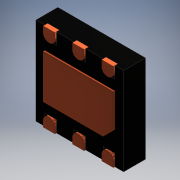
# Autodesk Inventor part: 3x3 6-pin DFN
Saved by Autodesk Inventor 2016 (Build 200138000, 138)
## iProperties
Created: 2016-07-18
Part Number: 3x3 6-pin DFN
Material: Generic
Document SubType Name: Modeling
Designer: Jonathan
Density: 1 g/cm^3
Appearance: Default
Author: Jonathan
Autodesk Inventor part; units mm, degrees
ref_plane "YZ Plane" through (0, 0, 0) normal (1, 0, 0) x (0, 1, 0)
ref_plane "XZ Plane" through (0, 0, 0) normal (0, 1, 0) x (-1, 0, 0)
ref_plane "XY Plane" through (0, 0, 0) normal (0, 0, 1) x (1, 0, 0)
sketch "Sketch1" plane through (0, 0, 0) normal (0, 1, 0) x (-1, 0, 0)
  line L0 (-1.5, 1.5) -> (1.5, 1.5)
  line L1 (1.5, 1.5) -> (1.5, -1.5)
  line L2 (1.5, -1.5) -> (-1.5, -1.5)
  line L3 (-1.5, -1.5) -> (-1.5, 1.5)
  line L4 (-1.5, 1.5) -> (1.5, -1.5) construction
  line L5 (1.5, 1.5) -> (-1.5, -1.5) construction
  point P0 (0, 0)
  dimension "d0" = 3
  dimension "d1" = 3
  constraints: 12 end point, 2 midpoint, 2 parallel, 1 horizontal, 1 perpendicular
  measures "d0" distance of L0.end L1.end
  measures "d1" distance of L0.start L0.end
extrude "Extrusion1" add sketch "Sketch1" along normal mid plane 0.75
sketch "Sketch3" plane through (0, -0.375, 0) normal (0, -1, 0) x (1, 0, 0)
  line L0 (-1.5, 1.5) -> (1.5, 1.5) projected
  line L1 (0.2, 1.5) -> (-0.2, 1.5)
  line L2 (-0.2, 1.5) -> (-0.2, 1.1)
  line L3 (-0.2, 1.1) -> (0.2, 1.1)
  line L4 (0.2, 1.1) -> (0.2, 1.5)
  point P0 (0, 0)
  point P1 (0, 1.1)
  dimension "d6" = 0.4
  dimension "d7" = 0.4
  constraints: 8 end point, 2 parallel, 1 horizontal, 1 midpoint, 1 perpendicular, 1 point on line, 1 vertical alignment
  measures "d6" distance of L3.end L1.start
  measures "d7" distance of L2.end L3.end
extrude "Extrusion2" cut sketch "Sketch3" against normal blind 0.1
sketch "Sketch4" plane through (0, -0.275, 0) normal (0, -1, 0) x (1, 0, 0)
  line L0 (-0.2, 1.1) -> (-0.2, 1.5) projected
  line L1 (0.2, 1.5) -> (-0.2, 1.5)
  line L2 (-0.2, 1.5) -> (-0.2, 1.4)
  line L3 (-0.2, 1.4) -> (0.2, 1.4)
  line L4 (0.2, 1.4) -> (0.2, 1.5)
  line L5 (0.2, 1.5) -> (0.2, 1.1) projected
  point P0 (0, 0)
  dimension "d10" = 0.1
  constraints: 8 end point, 2 parallel, 1 collinear, 1 horizontal, 1 perpendicular, 1 point on line
  measures "d10" distance of L3.end L1.start
extrude "Extrusion3" add sketch "Sketch4" along normal blind 0.15 separate body
sketch "Sketch6" plane through (0, -0.425, 0) normal (0, -1, 0) x (1, 0, 0)
  line L0 (-0.2, 1.4) -> (0.2, 1.4) projected
  line L1 (0.2, 1.4) -> (0.2, 1.3)
  line L2 (-0.2, 1.4) -> (-0.2, 1.3)
  line L3 (-0.2, 1.1) -> (-0.2, 1.5) projected
  arc A0 (-0.2, 1.3) -> (0.2, 1.3) centre (0, 1.3) ccw
  line L4 (0.25, 1.1) -> (-0.25, 1.1) construction
  line L5 (0.2, 1.1) -> (-0.2, 1.1) projected
  point P0 (0, 0)
  point P1 (0, 1.1)
  dimension "d13" = 0.5
  constraints: 6 end point, 3 point on circle, 2 midpoint, 2 tangent, 1 centre point, 1 collinear, 1 horizontal, 1 vertical
  measures "d13" distance of L4.start L4.end
extrude "Extrusion4" add sketch "Sketch6" against normal blind 0.1 contours L0 L1 A0 L2 bodies 2
pattern_linear "Rectangular Pattern1" count 2 spacing 1 along (-1, 0, 0) count 2 spacing 1 along (1, 0, 0) of "Extrusion2" bodies 1
pattern_linear "Rectangular Pattern2" count 2 spacing 1 along (-1, 0, 0) count 2 spacing 1 along (1, 0, 0) of "Extrusion3", "Extrusion4" bodies 2
mirror "Mirror1" about plane through (0, 0, 0) normal (0, 0, 1) of "Extrusion2", "Rectangular Pattern1" bodies 1
mirror "Mirror2" about plane through (0, 0, 0) normal (0, 0, 1) of "Extrusion3", "Extrusion4", "Rectangular Pattern2" bodies 2
sketch "Sketch7" plane through (0, -0.375, 0) normal (0, -1, 0) x (1, 0, 0)
  line L0 (-1.2, 0.75) -> (1.2, 0.75)
  line L1 (1.2, 0.75) -> (1.2, -0.3964)
  line L2 (0.8464, -0.75) -> (-1.2, -0.75)
  line L3 (-1.2, -0.75) -> (-1.2, 0.75)
  line L4 (-1.2, 0.75) -> (1.2, -0.75) construction
  line L5 (1.2, 0.75) -> (-1.2, -0.75) construction
  line L6 (1.2, -0.3964) -> (0.8464, -0.75)
  point P0 (0, 0)
  point P1 (-0.1768, -0.75)
  point P2 (1.2, 0.1768)
  dimension "d28" = 1.5
  dimension "d29" = 2.4
  dimension "d30" = 135
  dimension "d31" = 0.5
  constraints: 14 end point, 4 midpoint, 2 parallel, 1 horizontal, 1 horizontal alignment, 1 perpendicular, 1 vertical alignment
  measures "d28" distance between parallel lines of L2 L0
  measures "d29" distance of L0.start L0.end
  measures "d30" angle of L2 L6
  measures "d31" distance of L1.end L2.start
extrude "Extrusion5" cut sketch "Sketch7" against normal blind 0.01 bodies 1
extrude "Extrusion6" add sketch "Sketch7" along normal up to surface (0.05 mm away) bodies 2
sketch "Sketch8" plane through (0, 0.375, 0) normal (0, 1, 0) x (1, 0, 0)
  circle A0 centre (0, 0) radius 0.72
  dimension "d36" = 1.44
  constraints: 1 centre point, 1 coincident
  measures "d36" diameter of A0
sketch "Sketch9" plane through (0, 0, 0) normal (0, 1, 0) x (-1, 0, 0)
  circle A0 centre (0, 0) radius 0.45
  dimension "d37" = 0.9
  constraints: 1 centre point, 1 coincident
  measures "d37" diameter of A0
loft "Loft1" cut profiles "Sketch8", "Sketch9" bodies 1
sketch "Sketch10" plane through (0, 0.375, 0) normal (0, 1, 0) x (1, 0, 0)
  circle A0 centre (1.15, 1.15) radius 0.125
  line L0 (1.5, -1.5) -> (1.5, 1.5) projected
  line L1 (1.5, 1.5) -> (-1.5, 1.5) projected
  point P0 (0, 0)
  dimension "d42" = 0.25
  dimension "d43" = 0.35
  dimension "d44" = 0.35
  constraints: 1 centre point
  measures "d42" diameter of A0
  measures "d43" distance from line of L0 A0.centre
  measures "d44" distance from line of L1 A0.centre
extrude "Extrusion7" cut sketch "Sketch10" against normal blind 0.05 bodies 1
body "Solid1"
body "Solid2"
